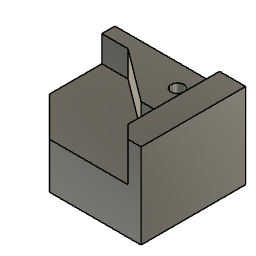
PIECE_1_robocon (Autodesk Fusion 360 design; units mm, degrees)
Autodesk Fusion 360 part; units mm, degrees
sketch "Sketch1" plane through (0, 0, 0) normal (0, 0, 1) x (1, 0, 0) in component "Component"
  line L0 (41.5, -17) -> (-41.5, -17)
  line L1 (-41.5, -17) -> (-41.5, 17)
  line L2 (-41.5, 17) -> (41.5, 17)
  line L3 (41.5, 17) -> (41.5, -17)
  line L4 (41.5, -17) -> (-41.5, 17) construction
  line L5 (-41.5, -17) -> (41.5, 17) construction
  dimension "d1" = 83
  dimension "d2" = 34
  constraint horizontal L0
  constraint perpendicular L0 L1
  constraint parallel L0 L2
  constraint parallel L1 L3
  constraint coincident L4 origin
  constraint coincident L5 origin
  measures "d1" distance of L1.end L2.end
  measures "d2" distance of L0.end L1.end
sketch "Sketch2" plane through (0, 0, 38) normal (0, 0, 1) x (-1, 0, 0) in component "Component"
  line L0 (-41.5, -17) -> (41.5, -17)
  line L1 (41.5, -17) -> (41.5, 17)
  line L2 (41.5, 17) -> (-41.5, 17)
  line L3 (-41.5, 17) -> (-41.5, -17)
  line L4 (37.5, 13) -> (-37.5, 13)
  line L5 (-37.5, 13) -> (-37.5, -13)
  line L6 (-37.5, -13) -> (37.5, -13)
  line L7 (37.5, -13) -> (37.5, 13)
  dimension "d5" = -4
sketch "Sketch3" plane through (0, 0, 0) normal (0, 0, 1) x (1, 0, 0) in component "Component"
  line L0 (10, 8) -> (-10, 8)
  line L1 (-10, 8) -> (-10, -8)
  line L2 (-10, -8) -> (10, -8)
  line L3 (10, -8) -> (10, 8)
  line L4 (10, 8) -> (-10, -8) construction
  line L5 (-10, 8) -> (10, -8) construction
  dimension "d12" = 20
  dimension "d13" = 16
  constraint horizontal L0
  constraint perpendicular L0 L1
  constraint parallel L0 L2
  constraint parallel L1 L3
  constraint coincident L4 origin
  constraint coincident L5 origin
  measures "d12" distance of L1.end L2.end
  measures "d13" distance of L0.end L1.end
extrude "Extrude3" add sketch "Sketch3" along normal blind 13 in component "Component"
sketch "Sketch4" plane through (0, 0, 13) normal (0, 0, 1) x (-1, 0, 0) in component "Component"
  line L0 (-10, 8) -> (-10, -8)
  line L1 (-10, -8) -> (10, -8)
  line L2 (10, -8) -> (10, 8)
  line L3 (10, 8) -> (-10, 8)
  line L4 (-10, 8) -> (-6, 8)
  line L5 (-6, 8) -> (-6, -8)
  dimension "d16" = 4
  constraint coincident L0.start L3.end
  constraint perpendicular L0 L4
  constraint coincident L1 L5.end
  constraint perpendicular L1 L5
  measures "d16" distance of L0.start L4.end
extrude "Extrude4" cut sketch "Sketch4" against normal blind 2 contours L1 L2 L3 L5 in component "Component"
sketch "Sketch5" plane through (0, 0, 11) normal (0, 0, 1) x (-1, 0, 0) in component "Component"
  line L0 (-6, 8) -> (-6, -8)
  line L1 (-6, -8) -> (10, -8)
  line L2 (10, -8) -> (10, 8)
  line L3 (10, 8) -> (-6, 8)
  line L4 (10, -8) -> (10, -6)
  line L5 (10, -6) -> (6, -6)
  line L6 (-6, -8) -> (-6, 0)
  line L7 (-6, 0) -> (-2, 0)
  line L8 (6, -6) -> (-2, 0)
  dimension "d19" = 2
  dimension "d20" = 4
  dimension "d21" = 8
  dimension "d22" = 4
  constraint coincident L1.end L2.start
  constraint perpendicular L1 L4
  constraint perpendicular L4 L5
  constraint coincident L0.end L1.start
  constraint perpendicular L1 L6
  constraint perpendicular L6 L7
  measures "d19" distance of L1.end L4.end
  measures "d20" distance of L4.end L5.end
  measures "d21" distance of L0.end L6.end
  measures "d22" distance of L6.end L7.end
extrude "Extrude5" cut sketch "Sketch5" against normal blind 4 contours L0 L2 L3 L5 L7 L8 in component "Component"
chamfer "Chamfer1" distance 2 angle 45 1 edges at (6, -8, 10) in component "Component"
chamfer "Chamfer2" distance 6 angle 45 1 edges at (-10, -8, 3.5) in component "Component"
sketch "Sketch6" plane through (6, 0, 0) normal (-1, 0, 0) x (0, -1, 0) in component "Component"
  line L0 (6, 7) -> (6, 13)
  line L1 (6, 13) -> (-8, 13)
  line L2 (-8, 13) -> (-8, 11)
  line L3 (-8, 11) -> (0, 11)
  line L4 (0, 11) -> (0, 7)
  line L5 (0, 7) -> (6, 7)
  circle A0 centre (3, 10) radius 1
  dimension "d27" = 2
  measures "d27" diameter of A0
extrude "Extrude6" cut sketch "Sketch6" against normal blind 2 contours A0 in component "Component"
sketch "Sketch7" plane through (0, 0, 11) normal (0, 0, 1) x (-1, 0, 0) in component "Component"
  line L0 (10, -6) -> (6, -6)
  line L1 (6, -6) -> (-2, 0)
  line L2 (-2, 0) -> (-6, 0)
  line L3 (-6, 0) -> (-6, -8)
  line L4 (-6, -8) -> (10, -8)
  line L5 (10, -8) -> (10, -6)
  circle A0 through (-2.0273, -4.5409, -11) (-3.5273, -3.6749, -11) (-3.5273, -5.4069, -11)
  circle A1 through (-2.0247, -4.5495, -11) (-3.5247, -3.6835, -11) (-3.5247, -5.4155, -11)
  dimension "d30" = 2
  dimension "d31" = 2
extrude "Extrude7" cut sketch "Sketch7" along normal blind 11 contours A0 A1 in plane through (0, 0, 0) normal (0, 0, 1) picked at (2.9031, 4.8538, 0) in component "Component"
component "Component" placed x (1, 0, 0) y (0, 1, 0) z (0, 0, 1) at (0, 0, 0)
